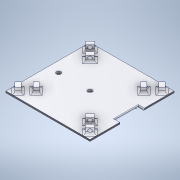
# Autodesk Inventor part: EM plate
Saved by Autodesk Inventor 2022 (Build 260153000, 153)
## iProperties
Created: 2022-02-15
Part Number: EM plate
Material: Steel, Cast
Document SubType Name: Modeling
Designer: Dahway
Density: 7.85 g/cm^3
Appearance: PTFE
Author: Dahway
Autodesk Inventor part; units mm, degrees
ref_plane "YZ Plane" through (0, 0, 0) normal (1, 0, 0) x (0, 1, 0)
ref_plane "XZ Plane" through (0, 0, 0) normal (0, 1, 0) x (-1, 0, 0)
ref_plane "XY Plane" through (0, 0, 0) normal (0, 0, 1) x (1, 0, 0)
sketch "Sketch1" plane through (0, 0, 0) normal (0, 1, 0) x (-1, 0, 0)
  line L0 (0, 0) -> (75, 0)
  line L1 (75, 0) -> (75, -75)
  line L2 (75, -75) -> (0, -75)
  line L3 (0, -75) -> (0, 0)
  dimension "d0" = 75
  dimension "d1" = 75
  constraints: 8 end point, 2 parallel, 1 horizontal, 1 perpendicular
  measures "d0" distance of L1.end L2.end
  measures "d1" distance of L0.end L1.end
extrude "Extrusion1" add sketch "Sketch1" along normal blind 3.5
sketch "Sketch4" plane through (0, 0, 0) normal (0, -1, 0) x (1, 0, 0)
  line L0 (0, -75) -> (-75, -75) projected
  line L1 (0, 0) -> (0, -75) projected
  point P0 (-37.5, -37.5)
  dimension "d22" = 37.5
  dimension "d23" = 37.5
  measures "d22" distance from line of L0 point (-37.5, -37.5)
  measures "d23" distance from line of L1 point (-37.5, -37.5)
hole "Hole2" at (-37.5, 0, -37.5) direction (0, 1, 0) diameter 4 end through all counterbore diameter 25.5 counterbore depth 1.5
chamfer "Chamfer1" distance 2 angle 45 4 edges at (0, 0, -37.5) (-37.5, 0, 0) (-37.5, 0, -75) (-75, 0, -37.5)
sketch "Sketch9" plane through (0, 0, 0) normal (0, -1, 0) x (1, 0, 0)
  circle A0 centre (-37.5, -37.5) radius 2 projected
  line L0 (-75, -75) -> (0, -75) projected
  point P0 (0, 0)
  point P1 (-65.5, -37.5)
  dimension "d89" = 28
  dimension "d90" = 37.5
  measures "d89" distance of A0.centre point (-65.5, -37.5)
  measures "d90" distance from line of L0 point (-65.5, -37.5)
hole "Hole5" at (-65.5, 0, -37.5) direction (0, 1, 0) diameter 4 end through all
sketch "Sketch11" plane through (0, 3.5, 0) normal (0, 1, 0) x (1, 0, 0)
  line L0 (-73, 2) -> (-2, 2) projected
  line L1 (-2, 2) -> (-2, 73) projected
  line L2 (-5.889, 2) -> (-2, 5.8892)
  line L3 (-2, 5.8892) -> (-4.8285, 8.7175)
  line L4 (-4.8285, 8.7175) -> (-8.7175, 4.8284)
  line L5 (-8.7175, 4.8284) -> (-5.889, 2)
  line L6 (-14.0209, 10.1315) -> (-10.1319, 14.0207)
  line L7 (-10.1319, 14.0207) -> (-12.9604, 16.8491)
  line L8 (-12.9604, 16.8491) -> (-16.8494, 12.9599)
  line L9 (-16.8494, 12.9599) -> (-14.0209, 10.1315)
  circle A0 centre (-37.5, 37.5) radius 2 projected
  point P0 (0, 0)
  dimension "d97" = 5.5
  dimension "d98" = 4
  dimension "d99" = 134.999
  dimension "d102" = 4
  dimension "d103" = 7.5
  dimension "d105" = 5.5
  dimension "d106" = 2.749
  constraints: 16 end point, 6 perpendicular, 2 point on line
  measures "d97" distance of L2.start L2.end
  measures "d98" distance of L2.end L3.end
  measures "d99" angle of L0 L2
  measures "d102" distance of L6.end L7.end
  measures "d103" distance between parallel lines of L4 L6
  measures "d105" distance between parallel lines of L9 L7
  measures "d106" distance from line of L7 A0.centre
extrude "Extrusion5" add sketch "Sketch11" along normal blind 5 contours L5 L4 L3 L2 | L9 L8 L7 L6
fillet "Fillet3" radius 2 8 edges at (-11.5462, 3.5, -15.4349) (-3.4142, 3.5, -7.3034) (-7.3032, 3.5, -3.4142) (-6.773, 3.5, -6.773) (-15.4352, 3.5, -11.5457) (-14.9049, 3.5, -14.9045) (-12.0764, 3.5, -12.0761) (-3.9445, 3.5, -3.9446)
sketch "Sketch13" plane through (-10.1319, 5.5, -14.0207) normal (0.7071227, 0, 0.7070909) x (0.7070909, 0, -0.7071227)
  line L0 (0, 0) -> (0, 3) projected
  line L1 (-5.5, 3) -> (0, 3) projected
  point P0 (-2.7502, -5.5)
  point P1 (-2.75, 1)
  dimension "d124" = 2.75
  dimension "d125" = 2
  measures "d124" distance from line of point (-2.75, 1) L0
  measures "d125" distance from line of L1 point (-2.75, 1)
hole "Hole7" at (-12.0764, 6.5, -12.0761) direction (-0.7071227, 0, -0.7070909) diameter 3 end through all both
pattern_circular "Circular Pattern6" count 4 over 360 about axis through (-37.5, 106.1237, -37.5) along (0, -1, 0) of "Extrusion5", "Fillet3", "Hole7"
sketch "Sketch14" plane through (0, 0, 0) normal (0, -1, 0) x (1, 0, 0)
  line L0 (0, -25) -> (-22, -25)
  line L1 (-22, -25) -> (-22, -50)
  line L2 (-22, -50) -> (0, -50)
  line L3 (0, -50) -> (0, -25)
  line L4 (0, 0) -> (-75, 0) projected
  line L5 (0, -75) -> (0, 0) projected
  circle A0 centre (-19.5, -27) radius 0.55
  circle A1 centre (-19.5, -48) radius 0.55
  circle A2 centre (-7, -27) radius 0.55
  circle A3 centre (-7, -48) radius 0.55
  dimension "d132" = 22
  dimension "d133" = 25
  dimension "d134" = 25
  dimension "d135" = 1.1
  dimension "d136" = 2
  dimension "d137" = 2.5
  dimension "d140" = 21
  dimension "d143" = 12.5
  constraints: 8 end point, 4 centre point, 2 horizontal, 2 parallel, 1 collinear, 1 perpendicular, 1 vertical, 6 other
  measures "d132" distance of L2.end L1.end
  measures "d133" distance of L1.end L0.end
  measures "d134" distance between parallel lines of L4 L0
  measures "d135" diameter of A0
  measures "d136" distance from line of L0 A0.centre
  measures "d137" distance from line of L1 A0.centre
  measures "d140" distance of A0.centre A1.centre
  measures "d143" distance of A0.centre A2.centre
extrude "Extrusion6" cut sketch "Sketch14" against normal blind 2
sketch "Sketch15" plane through (0, 2, 0) normal (0, -1, 0) x (1, 0, 0)
  line L0 (0, -6.7176) -> (0, -68.2826) projected
  line L1 (0, -26.5) -> (-5, -26.5)
  line L2 (-5, -26.5) -> (-5, -48.5)
  line L3 (-5, -48.5) -> (0, -48.5)
  line L4 (0, -48.5) -> (0, -26.5)
  line L5 (0, -50) -> (-2, -50) projected
  point P0 (0, 0)
  point P1 (0, -48.5)
  dimension "d148" = 5
  dimension "d149" = 22
  dimension "d150" = 1.5
  constraints: 8 end point, 2 parallel, 1 horizontal, 1 perpendicular, 1 point on line
  measures "d148" distance of L3.end L2.end
  measures "d149" distance of L2.end L1.end
  measures "d150" distance between parallel lines of L5 L3
extrude "Extrusion7" cut sketch "Sketch15" against normal up to surface (1.5 mm away)
fillet "Fillet4" radius 0.5 2 edges at (-5, 2, -37.5) (-5, 3.5, -37.5)
fillet "Fillet5" radius 0.5 4 edges at (-7.55, 2, -27) (-20.05, 2, -27) (-20.05, 2, -48) (-7.55, 2, -48)
body "Solid1"
